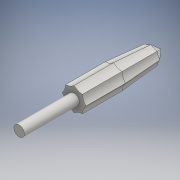
# Autodesk Inventor part: mixer
Saved by Autodesk Inventor 2016 (Build 200138000, 138)
## iProperties
Created: 2017-01-26
Part Number: mixer
Material: PBT Plastic
Document SubType Name: Modeling
Designer: Teta
Density: 1.31 g/cm^3
Appearance: Smooth - White
Author: Teta
Autodesk Inventor part; units mm, degrees
sketch "Sketch1" plane through (0, 0, 0) normal (1, 0, 0) x (0, 1, 0)
  point P0 (0, 0)
sketch "Sketch2" plane through (0, 0, 0) normal (0, 1, 0) x (-1, 0, 0)
  circle A0 centre (0, 0) radius 2
  dimension "d0" = 4
  constraints: 1 centre point, 1 coincident
  measures "d0" diameter of A0
extrude "Extrusion1" add sketch "Sketch2" along normal blind 25.2
sketch "Sketch3" plane through (0, 25.2, 0) normal (0, 1, 0) x (1, 0, 0)
  circle A0 centre (0, 0) radius 2 projected
  circle A1 centre (0, 0) radius 4.5
  dimension "d3" = 9
  constraints: 1 centre point, 1 coincident
  measures "d3" diameter of A1
extrude "Extrusion2" add sketch "Sketch3" along normal blind 2 contours A0 | A1
sketch "Sketch4" plane through (0, 27.2, 0) normal (0, 1, 0) x (1, 0, 0)
  circle A0 centre (0, 0) radius 4.5 projected
extrude "Extrusion3" add sketch "Sketch4" along normal blind 8.5
sketch "Sketch5" plane through (0, 35.7, 0) normal (0, 1, 0) x (1, 0, 0)
  point P0 (0, 0)
ref_plane "Work Plane1" through (0, 49.8, 0) normal (0, 1, 0) x (1, 0, 0)
sketch "Sketch6" plane through (0, 49.8, 0) normal (0, 1, 0) x (1, 0, 0)
  arc A0 (2.3688, -2.3688) -> (0, -3.35) centre (3.0339, -7.3244) ccw
  arc A1 (0, -3.35) -> (-2.3688, -2.3688) centre (-3.0339, -7.3244) ccw
  arc A2 (3.35, 0) -> (2.3688, -2.3688) centre (7.3244, -3.0339) ccw
  arc A3 (2.3688, 2.3688) -> (3.35, 0) centre (7.3244, 3.0339) ccw
  arc A4 (-3.35, 0) -> (-2.3688, 2.3688) centre (-7.3244, 3.0339) ccw
  arc A5 (-2.3688, -2.3688) -> (-3.35, 0) centre (-7.3244, -3.0339) ccw
  arc A6 (-2.3688, 2.3688) -> (0, 3.35) centre (-3.0339, 7.3244) ccw
  arc A7 (0, 3.35) -> (2.3688, 2.3688) centre (3.0339, 7.3244) ccw
  point P0 (0, 0)
  dimension "d25" = 5
  constraints: 16 point on circle, 8 centre point
  measures "d25" radius of A0
sketch "Sketch7" plane through (0, 35.7, 0) normal (0, 1, 0) x (1, 0, 0)
  circle A0 centre (0, 0) radius 4.5 projected
  circle A1 centre (0, 0) radius 4.5 projected
  arc A2 (-3.1879, -3.176) -> (-4.5, 0.0084) centre (-8.1841, -3.372) ccw
  arc A3 (-4.5, 0.0084) -> (-3.176, 3.1879) centre (-8.1714, 3.4027) ccw
  arc A4 (4.5, -0.0084) -> (3.176, -3.1879) centre (8.1714, -3.4027) ccw
  arc A5 (3.1879, 3.176) -> (4.5, -0.0084) centre (8.1841, 3.372) ccw
  arc A6 (-0.0084, -4.5) -> (-3.1879, -3.176) centre (-3.4027, -8.1714) ccw
  arc A7 (3.176, -3.1879) -> (-0.0084, -4.5) centre (3.372, -8.1841) ccw
  arc A8 (0.0084, 4.5) -> (3.1879, 3.176) centre (3.4027, 8.1714) ccw
  arc A9 (-3.176, 3.1879) -> (0.0084, 4.5) centre (-3.372, 8.1841) ccw
  circle A10 centre (0, 0) radius 4.5
  constraints: 16 point on circle, 8 centre point, 7 other
extrude "Extrusion4" cut sketch "Sketch7" against normal blind 8.5 contours A0 A5 | A8 A0 | A0 A4 | A9 A0 | A0 A7 | A3 A0 | A0 A6 | A2 A0
ref_plane "Work Plane2" through (0, 49.8, 0) normal (0, 1, 0) x (1, 0, 0)
loft "Loft2" add profiles "Sketch6" section 2 edges at (-1.4806, 35.7, 3.5556) (1.4672, 35.7, 3.5611) (3.5556, 35.7, 1.4806) (3.5611, 35.7, -1.4672) (1.4806, 35.7, -3.5556) (-1.4672, 35.7, -3.5611) (-3.5556, 35.7, -1.4806) (-3.5611, 35.7, 1.4672)
sketch "Sketch10" plane through (0, 27.2, 0) normal (0, 1, 0) x (1, 0, 0)
  arc A0 (3.176, -3.1879) -> (-0.0084, -4.5) centre (3.372, -8.1841) ccw projected
  arc A1 (-0.0084, -4.5) -> (3.176, -3.1879) centre (0, 0) ccw projected
  arc A2 (-0.0084, -4.5) -> (-3.1879, -3.176) centre (-3.4027, -8.1714) ccw projected
  arc A3 (-0.0084, -4.5) -> (-3.1879, -3.176) centre (-3.4027, -8.1714) ccw projected
  arc A4 (-3.1879, -3.176) -> (-0.0084, -4.5) centre (0, 0) ccw projected
  arc A5 (-3.1879, -3.176) -> (-4.5, 0.0084) centre (-8.1841, -3.372) ccw projected
  arc A6 (-4.5, 0.0084) -> (-3.1879, -3.176) centre (0, 0) ccw projected
  arc A7 (-4.5, 0.0084) -> (-3.176, 3.1879) centre (-8.1714, 3.4027) ccw projected
  arc A8 (-3.176, 3.1879) -> (-4.5, 0.0084) centre (0, 0) ccw projected
  arc A9 (-3.176, 3.1879) -> (0.0084, 4.5) centre (-3.372, 8.1841) ccw projected
  arc A10 (-3.176, 3.1879) -> (0.0084, 4.5) centre (-3.372, 8.1841) ccw projected
  arc A11 (0.0084, 4.5) -> (-3.176, 3.1879) centre (0, 0) ccw projected
  arc A12 (0.0084, 4.5) -> (3.1879, 3.176) centre (3.4027, 8.1714) ccw projected
  arc A13 (3.1879, 3.176) -> (0.0084, 4.5) centre (0, 0) ccw projected
  arc A14 (3.1879, 3.176) -> (4.5, -0.0084) centre (8.1841, 3.372) ccw projected
  arc A15 (4.5, -0.0084) -> (3.1879, 3.176) centre (0, 0) ccw projected
  arc A16 (4.5, -0.0084) -> (3.176, -3.1879) centre (8.1714, -3.4027) ccw projected
  arc A17 (3.176, -3.1879) -> (4.5, -0.0084) centre (0, 0) ccw projected
extrude "Extrusion5" cut sketch "Sketch10" against normal blind 10 contours A1 A0 | A16 A17 | A4 A2 | A14 A15 | A6 A5 | A12 A13 | A8 A7 | A9 A11
sketch "Sketch11" plane through (0, 25.2, 0) normal (0, -1, 0) x (1, 0, 0)
  point P0 (0, 0)
ref_plane "Work Plane3" through (0, 20.75, 0) normal (0, -1, 0) x (1, 0, 0)
sketch "Sketch12" plane through (0, 20.75, 0) normal (0, -1, 0) x (1, 0, 0)
  circle A0 centre (0, 0) radius 2 projected
  circle A1 centre (0, 0) radius 3.5
  dimension "d33" = 7
  constraints: 1 centre point, 1 coincident
  measures "d33" diameter of A1
extrude "Extrusion6" add sketch "Sketch12" against normal blind 1
fillet "Fillet1" radius 0.5 1 edges at (-3.5, 21.75, 0)
sketch "Sketch13" plane through (0, 20.75, 0) normal (0, -1, 0) x (1, 0, 0)
  arc A0 (3.176, 3.1879) -> (4.5, 0.0084) centre (8.1714, 3.4027) ccw projected
  arc A1 (-0.0084, 4.5) -> (3.176, 3.1879) centre (3.372, 8.1841) ccw projected
  arc A2 (-3.1879, 3.176) -> (-0.0084, 4.5) centre (-3.4027, 8.1714) ccw projected
  arc A3 (-4.5, -0.0084) -> (-3.1879, 3.176) centre (-8.1841, 3.372) ccw projected
  arc A4 (-3.176, -3.1879) -> (-4.5, -0.0084) centre (-8.1714, -3.4027) ccw projected
  arc A5 (0.0084, -4.5) -> (-3.176, -3.1879) centre (-3.372, -8.1841) ccw projected
  arc A6 (3.1879, -3.176) -> (0.0084, -4.5) centre (3.4027, -8.1714) ccw projected
  arc A7 (4.5, 0.0084) -> (3.1879, -3.176) centre (8.1841, -3.372) ccw projected
  circle A8 centre (0, 0) radius 2 projected
extrude "Extrusion7" add sketch "Sketch13" against normal blind 10
ref_plane "Work Plane4" through (3.0339, 53.55, 7.3244) normal (0, 1, 0) x (0.9238795, 0, -0.3826834)
sketch "Sketch16" plane through (3.0339, 53.55, 7.3244) normal (0, 1, 0) x (0.9238795, 0, -0.3826834)
  arc A0 (1.282, 4.8329) -> (-1.282, 4.8329) centre (0, 0) ccw projected
  arc A1 (3.095, 6.6459) -> (1.282, 4.8329) centre (5.6058, 2.322) ccw projected
  arc A2 (3.095, 9.2098) -> (3.095, 6.6459) centre (7.9279, 7.9279) ccw projected
  arc A3 (1.282, 11.0228) -> (3.095, 9.2098) centre (5.6058, 13.5337) ccw projected
  arc A4 (-1.282, 11.0228) -> (1.282, 11.0228) centre (0, 15.8557) ccw projected
  arc A5 (-3.095, 9.2098) -> (-1.282, 11.0228) centre (-5.6058, 13.5337) ccw projected
  arc A6 (-3.095, 6.6459) -> (-3.095, 9.2098) centre (-7.9279, 7.9279) ccw projected
  arc A7 (-1.282, 4.8329) -> (-3.095, 6.6459) centre (-5.6058, 2.322) ccw projected
  point P0 (0, 7.9279)
  point P1 (0, 7.9279)
  constraints: 1 coincident
loft "Loft4" add section 1 edges at (1.1204, 49.8, 2.705) (2.705, 49.8, 1.1204) (2.705, 49.8, -1.1204) (1.1204, 49.8, -2.705) (-1.1204, 49.8, -2.705) (-2.705, 49.8, -1.1204) (-2.705, 49.8, 1.1204) (-1.1204, 49.8, 2.705) section 2 point at (0, 53.55, 0)
body "Solid1"
